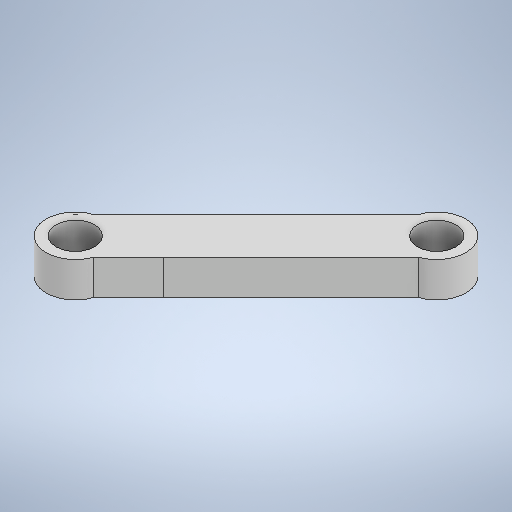
# Autodesk Inventor part: LINKV2
Saved by Autodesk Inventor 2025.1 (Build 291241000, 241)
## iProperties
Created: 2024-10-27
Part Number: LINKV2
Material: Generic
Document SubType Name: Modeling
Designer: m_kni
Density: 1 g/cm^3
Appearance: Default
Author: m_kni
Autodesk Inventor part; units mm, degrees
ref_plane "YZ Plane" through (0, 0, 0) normal (1, 0, 0) x (0, 1, 0)
ref_plane "XZ Plane" through (0, 0, 0) normal (0, 1, 0) x (-1, 0, 0)
ref_plane "XY Plane" through (0, 0, 0) normal (0, 0, 1) x (1, 0, 0)
sketch "Sketch1" plane through (0, 0, 0) normal (0, 1, 0) x (-1, 0, 0)
  arc A0 (-7.7903, -4.6284) -> (-4.6931, -7.8909) centre (-6.2844, -6.3003) ccw
  arc A1 (-7.7903, -4.6284) -> (-4.6931, -7.8909) centre (-6.2844, -6.3003) ccw
  circle A2 centre (9.2097, 9.1939) radius 1.65
  circle A3 centre (-6.2844, -6.3003) radius 1.65
  arc A4 (-7.7903, -4.6284) -> (-4.6931, -7.8909) centre (-6.2844, -6.3003) ccw
  line L0 (3.8206, 6.9818) -> (-7.7903, -4.6284)
  line L1 (7.2787, 10.4444) -> (3.8206, 6.9818)
  arc A5 (7.3269, 10.4258) -> (7.2787, 10.4444) centre (5.3206, 5.3048) ccw
  arc A6 (10.8867, 7.6938) -> (7.3269, 10.4258) centre (9.2097, 9.1939) ccw
  line L2 (10.7098, 7.5169) -> (10.8867, 7.6938)
  arc A7 (10.4416, 7.3111) -> (10.7098, 7.5169) centre (9.2097, 9.1939) ccw
  arc A8 (10.459, 7.2661) -> (10.4416, 7.3111) centre (5.3206, 5.3048) ccw
  line L3 (6.9976, 3.8047) -> (10.459, 7.2661)
  line L4 (-4.6931, -7.8909) -> (6.9976, 3.8047)
  circle A9 centre (-6.2844, -6.3003) radius 1.75
  arc A10 (-7.7903, -4.6284) -> (-4.6931, -7.8909) centre (-6.2844, -6.3003) ccw
  line L5 (-4.6931, -7.8909) -> (6.9976, 3.8047)
  line L6 (6.9976, 3.8047) -> (10.459, 7.2661)
  arc A11 (10.459, 7.2661) -> (10.4416, 7.3111) centre (5.3206, 5.3048) ccw
  arc A12 (10.4416, 7.3111) -> (10.7098, 7.5169) centre (9.2097, 9.1939) ccw
  line L7 (10.7098, 7.5169) -> (10.8867, 7.6938)
  arc A13 (10.8867, 7.6938) -> (7.3269, 10.4258) centre (9.2097, 9.1939) ccw
  arc A14 (7.3269, 10.4258) -> (7.2787, 10.4444) centre (5.3206, 5.3048) ccw
  line L8 (7.2787, 10.4444) -> (3.8206, 6.9818)
  line L9 (3.8206, 6.9818) -> (-7.7903, -4.6284)
  line L10 (3.8206, 6.9818) -> (-7.7903, -4.6284)
  line L11 (3.8206, 6.9818) -> (-7.7903, -4.6284)
  line L12 (3.8206, 6.9818) -> (-7.7903, -4.6284)
  line L13 (3.8206, 6.9818) -> (-7.7903, -4.6284)
  line L14 (-4.6931, -7.8909) -> (6.9976, 3.8047)
  line L15 (-4.6931, -7.8909) -> (6.9976, 3.8047)
  line L16 (-4.6931, -7.8909) -> (6.9976, 3.8047)
  line L17 (-4.6931, -7.8909) -> (6.9976, 3.8047)
  circle A15 centre (-6.2844, -6.3003) radius 1.75
  circle A16 centre (-6.2844, -6.3003) radius 1.75
  circle A17 centre (-6.2844, -6.3003) radius 1.75
  circle A18 centre (-6.2844, -6.3003) radius 1.75
  arc A19 (-7.7903, -4.6284) -> (-4.6931, -7.8909) centre (-6.2844, -6.3003) ccw
  arc A20 (-7.7903, -4.6284) -> (-4.6931, -7.8909) centre (-6.2844, -6.3003) ccw
  line L18 (7.2787, 10.4444) -> (3.8206, 6.9818)
  line L19 (7.2787, 10.4444) -> (3.8206, 6.9818)
  line L20 (7.2787, 10.4444) -> (3.8206, 6.9818)
  line L21 (7.2787, 10.4444) -> (3.8206, 6.9818)
  line L22 (6.9976, 3.8047) -> (10.459, 7.2661)
  line L23 (6.9976, 3.8047) -> (10.459, 7.2661)
  line L24 (6.9976, 3.8047) -> (10.459, 7.2661)
  line L25 (6.9976, 3.8047) -> (10.459, 7.2661)
  arc A21 (7.3269, 10.4258) -> (7.2787, 10.4444) centre (5.3206, 5.3048) ccw
  arc A22 (7.3269, 10.4258) -> (7.2787, 10.4444) centre (5.3206, 5.3048) ccw
  arc A23 (10.459, 7.2661) -> (10.4416, 7.3111) centre (5.3206, 5.3048) ccw
  arc A24 (10.459, 7.2661) -> (10.4416, 7.3111) centre (5.3206, 5.3048) ccw
  arc A25 (10.459, 7.2661) -> (10.4416, 7.3111) centre (5.3206, 5.3048) ccw
  arc A26 (10.459, 7.2661) -> (10.4416, 7.3111) centre (5.3206, 5.3048) ccw
  arc A27 (10.4416, 7.3111) -> (10.7098, 7.5169) centre (9.2097, 9.1939) ccw
  arc A28 (10.4416, 7.3111) -> (10.7098, 7.5169) centre (9.2097, 9.1939) ccw
  arc A29 (10.4416, 7.3111) -> (10.7098, 7.5169) centre (9.2097, 9.1939) ccw
  arc A30 (10.4416, 7.3111) -> (10.7098, 7.5169) centre (9.2097, 9.1939) ccw
  line L26 (10.7098, 7.5169) -> (10.8867, 7.6938)
  line L27 (10.7098, 7.5169) -> (10.8867, 7.6938)
  arc A31 (7.3269, 10.4258) -> (7.2787, 10.4444) centre (5.3206, 5.3048) ccw
  line L28 (10.7098, 7.5169) -> (10.8867, 7.6938)
  arc A32 (10.8867, 7.6938) -> (7.3269, 10.4258) centre (9.2097, 9.1939) ccw
  arc A33 (10.8867, 7.6938) -> (7.3269, 10.4258) centre (9.2097, 9.1939) ccw
  arc A34 (10.8867, 7.6938) -> (7.3269, 10.4258) centre (9.2097, 9.1939) ccw
  arc A35 (10.8867, 7.6938) -> (7.3269, 10.4258) centre (9.2097, 9.1939) ccw
  line L29 (10.7098, 7.5169) -> (10.8867, 7.6938)
  circle A36 centre (9.2097, 9.1939) radius 1.75
  arc A37 (7.3269, 10.4258) -> (7.2787, 10.4444) centre (5.3206, 5.3048) ccw
  circle A38 centre (-6.2844, -6.3003) radius 1.75
  circle A39 centre (-6.2844, -6.3003) radius 2.5
  circle A40 centre (9.2097, 9.1939) radius 2.5
  circle A41 centre (-6.2844, -6.3003) radius 2.5
  circle A42 centre (9.2097, 9.1939) radius 2.25
  point P0 (0, 0)
  point P1 (-12.3012, -12.317)
  point P2 (10.0226, 6.8297)
  point P3 (6.8476, 10.0128)
  point P4 (-7.0982, -3.9364)
  point P5 (-3.9227, -7.1202)
  dimension "d0" = 5
  dimension "d1" = 5
  dimension "d4" = 3.3
  dimension "d5" = 3.3
  constraints: 56 end point, 56 point on circle, 41 centre point, 4 coincident, 3 concentric, 14 other
  measures "d0" diameter of A39
  measures "d1" diameter of A40
  measures "d4" diameter of A2
  measures "d5" diameter of A3
extrude "Extrusion1" add sketch "Sketch1" along normal blind 3 contours L0 A39 L4 A0 | A0 L4 A39 L0 | L0 L1 A40 L3 L4 A39 | A40 L3 A8 A7 A42 A6 A5 L1 | L1 A5 A42 A8 L3 A40 | A6 L2 A7 A42 | A9 | A36
body "Solid1"
